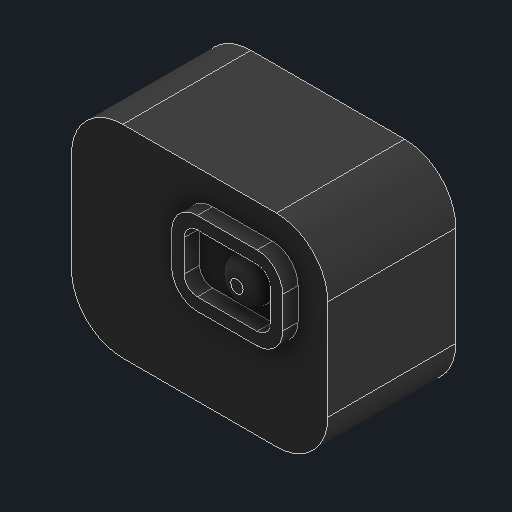
# Autodesk Inventor part: temp camera
Saved by Autodesk Inventor 2026.2 (Build 302298000, 298)
## iProperties
Created: 2025-12-19
Part Number: temp camera
Material: Rubber
Document SubType Name: Modeling
Designer: colin
Density: 0.93 g/cm^3
Appearance: Rubber - Black
Author: colin
Autodesk Inventor part; units mm, degrees
ref_plane "YZ Plane" through (0, 0, 0) normal (1, 0, 0) x (0, 1, 0)
ref_plane "XZ Plane" through (0, 0, 0) normal (0, 1, 0) x (-1, 0, 0)
ref_plane "XY Plane" through (0, 0, 0) normal (0, 0, 1) x (1, 0, 0)
sketch "Sketch1" plane through (0, 0, 0) normal (0, 0, 1) x (1, 0, 0)
  line L0 (10, 0) -> (40, 0)
  line L1 (50, 10) -> (50, 29.4958)
  line L2 (40, 39.4958) -> (10, 39.4958)
  line L3 (0, 29.4958) -> (0, 10)
  arc A0 (10, 39.4958) -> (0, 29.4958) centre (10, 29.4958) ccw
  arc A1 (50, 29.4958) -> (40, 39.4958) centre (40, 29.4958) ccw
  arc A2 (40, 0) -> (50, 10) centre (40, 10) ccw
  arc A3 (0, 10) -> (10, 0) centre (10, 10) ccw
  point P0 (0, 0)
  point P1 (50, 39.4958)
  point P2 (0, 39.4958)
  dimension "d0" = 50
  dimension "d1" = 10
  constraints: 8 end point, 8 point on circle, 8 tangent, 6 point on line, 4 centre point, 3 equal radius, 2 parallel, 1 horizontal, 1 perpendicular
  measures "d0" distance of point (0, 39.496) point (50, 39.496)
  measures "d1" radius of A0
extrude "Extrusion1" add sketch "Sketch1" along normal blind 25
sketch "Sketch2" plane through (0, 0, 25) normal (0, 0, 1) x (1, 0, 0)
  line L0 (39.1979, 34.3605) -> (27.5461, 34.3605)
  line L1 (22.5461, 29.3605) -> (22.5461, 23.1687)
  line L2 (27.5461, 18.1687) -> (39.1979, 18.1687)
  line L3 (44.1979, 23.1687) -> (44.1979, 29.3605)
  arc A0 (27.5461, 34.3605) -> (22.5461, 29.3605) centre (27.5461, 29.3605) ccw
  arc A1 (44.1979, 29.3605) -> (39.1979, 34.3605) centre (39.1979, 29.3605) ccw
  arc A2 (39.1979, 18.1687) -> (44.1979, 23.1687) centre (39.1979, 23.1687) ccw
  arc A3 (22.5461, 23.1687) -> (27.5461, 18.1687) centre (27.5461, 23.1687) ccw
  line L4 (27.5461, 31.9141) -> (39.1979, 31.9141)
  arc A4 (41.7515, 29.3605) -> (39.1979, 31.9141) centre (39.1979, 29.3605) ccw
  line L5 (41.7515, 29.3605) -> (41.7515, 23.1687)
  arc A5 (39.1979, 20.6151) -> (41.7515, 23.1687) centre (39.1979, 23.1687) ccw
  line L6 (39.1979, 20.6151) -> (27.5461, 20.6151)
  arc A6 (24.9925, 23.1687) -> (27.5461, 20.6151) centre (27.5461, 23.1687) ccw
  line L7 (24.9925, 23.1687) -> (24.9925, 29.3605)
  arc A7 (27.5461, 31.9141) -> (24.9925, 29.3605) centre (27.5461, 29.3605) ccw
  circle A8 centre (35.2717, 26.2646) radius 4.2058
  point P0 (0, 0)
  dimension "d4" = 5
  constraints: 16 end point, 16 point on circle, 9 centre point, 8 tangent, 4 parallel, 3 equal radius, 2 perpendicular, 1 horizontal, 7 other
  measures "d4" radius of A0
extrude "Extrusion2" add sketch "Sketch2" along normal blind 3
fillet "Fillet1" radius 3 1 edges at (31.0659, 26.2646, 28)
sketch "Sketch3" plane through (10, 0, 0) normal (0, -1, 0) x (1, 0, 0)
  circle A0 centre (14.5059, 11.6029) radius 2.3072
  point P0 (-10, 0)
  constraints: 1 centre point
extrude "Extrusion3" add sketch "Sketch3" along normal blind 1
body "Solid1"
